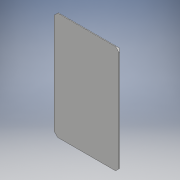
# Autodesk Inventor part: Деталь1
Saved by Autodesk Inventor 2018.1 (Build 221171000, 171)
## iProperties
Created: 2023-03-20
Part Number: Деталь1
Material: Типовые
Document SubType Name: Modeling
Designer: student
Density: 1 g/cm^3
Appearance: По умолчанию
Author: student
Autodesk Inventor part; units mm, degrees
ref_plane "YZ Plane" through (0, 0, 0) normal (1, 0, 0) x (0, 1, 0)
ref_plane "XZ Plane" through (0, 0, 0) normal (0, 1, 0) x (-1, 0, 0)
ref_plane "XY Plane" through (0, 0, 0) normal (0, 0, 1) x (1, 0, 0)
sketch "Эскиз1" plane through (0, 0, 0) normal (0, 1, 0) x (-1, 0, 0)
  line L0 (0, 0) -> (95, 0)
  line L1 (95, 0) -> (95, -158)
  line L2 (95, -158) -> (0, -158)
  line L3 (0, -158) -> (0, 0)
  dimension "d0" = 95
  dimension "d1" = 158
  constraints: 8 end point, 2 parallel, 1 horizontal, 1 perpendicular
  measures "d0" distance of L1.end L2.end
  measures "d1" distance of L0.end L1.end
extrude "Выдавливание1" add sketch "Эскиз1" along normal blind 10
chamfer "Фаска1" distance 9 angle 45 1 edges at (0, 10, -79)
chamfer "Фаска2" distance 9 angle 45 1 edges at (-52, 10, 0)
chamfer "Фаска3" distance 9 angle 45 1 edges at (-52, 10, -158)
chamfer "Фаска4" distance 9 angle 45 1 edges at (-95, 10, -79)
chamfer "Фаска5" distance 5 angle 45 1 edges at (0, 0.5, 0)
chamfer "Фаска6" distance 5 angle 45 1 edges at (-95, 0.5, 0)
chamfer "Фаска7" distance 5 angle 45 1 edges at (-95, 0.5, -158)
chamfer "Фаска8" distance 5 angle 45 1 edges at (0, 0.5, -158)
